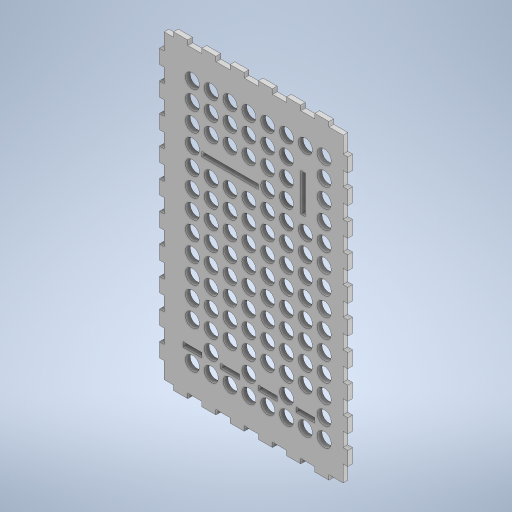
# Autodesk Inventor part: BackFrontPannel
Saved by Autodesk Inventor 2023 (Build 270158000, 158)
## iProperties
Created: 2022-09-19
Part Number: BackFrontPannel
Material: Generic
Document SubType Name: Modeling
Designer: Nathann
Density: 1 g/cm^3
Appearance: Default
Author: Nathann
Autodesk Inventor part; units mm, degrees
ref_plane "YZ Plane" through (0, 0, 0) normal (1, 0, 0) x (0, 1, 0)
ref_plane "XZ Plane" through (0, 0, 0) normal (0, 1, 0) x (-1, 0, 0)
ref_plane "XY Plane" through (0, 0, 0) normal (0, 0, 1) x (1, 0, 0)
sketch "Sketch1" plane through (0, 0, 0) normal (0, 0, 1) x (1, 0, 0)
  line L0 (0, 0) -> (200, 0)
  line L1 (200, 0) -> (200, -330)
  line L2 (200, -330) -> (0, -330)
  line L3 (0, -330) -> (0, 0)
  dimension "d0" = 200
  dimension "d1" = 330
  constraints: 8 end point, 2 parallel, 1 horizontal, 1 perpendicular
  measures "d0" distance of L0.start L0.end
  measures "d1" distance of L2.end L0.start
extrude "Extrusion1" add sketch "Sketch1" along normal blind 5
sketch "Sketch2" plane through (0, 0, 0) normal (0, 0, -1) x (-1, 0, 0)
  line L0 (0, 0) -> (-5, 0)
  line L1 (-5, 0) -> (-5, -22.5)
  line L2 (-5, -22.5) -> (0, -22.5)
  line L3 (0, -22.5) -> (0, 0)
  line L4 (-200, 0) -> (0, 0) projected
  line L5 (0, 0) -> (0, -330) projected
  line L6 (0, -37.5) -> (-5, -37.5)
  line L7 (-5, -37.5) -> (-5, -52.5)
  line L8 (-5, -52.5) -> (0, -52.5)
  line L9 (0, -52.5) -> (0, -37.5)
  line L10 (0, -30) -> (-5, -30)
  line L11 (0, -67.5) -> (-5, -67.5)
  line L12 (-5, -67.5) -> (-5, -82.5)
  line L13 (-5, -82.5) -> (0, -82.5)
  line L14 (0, -82.5) -> (0, -67.5)
  line L15 (0, -60) -> (-5, -60)
  line L16 (0, -97.5) -> (-5, -97.5)
  line L17 (-5, -97.5) -> (-5, -112.5)
  line L18 (-5, -112.5) -> (0, -112.5)
  line L19 (0, -112.5) -> (0, -97.5)
  line L20 (0, -90) -> (-5, -90)
  line L21 (0, -127.5) -> (-5, -127.5)
  line L22 (-5, -127.5) -> (-5, -142.5)
  line L23 (-5, -142.5) -> (0, -142.5)
  line L24 (0, -142.5) -> (0, -127.5)
  line L25 (0, -120) -> (-5, -120)
  line L26 (0, -157.5) -> (-5, -157.5)
  line L27 (-5, -157.5) -> (-5, -172.5)
  line L28 (-5, -172.5) -> (0, -172.5)
  line L29 (0, -172.5) -> (0, -157.5)
  line L30 (0, -150) -> (-5, -150)
  line L31 (0, -187.5) -> (-5, -187.5)
  line L32 (-5, -187.5) -> (-5, -202.5)
  line L33 (-5, -202.5) -> (0, -202.5)
  line L34 (0, -202.5) -> (0, -187.5)
  line L35 (0, -180) -> (-5, -180)
  line L36 (0, -217.5) -> (-5, -217.5)
  line L37 (-5, -217.5) -> (-5, -232.5)
  line L38 (-5, -232.5) -> (0, -232.5)
  line L39 (0, -232.5) -> (0, -217.5)
  line L40 (0, -210) -> (-5, -210)
  line L41 (0, -247.5) -> (-5, -247.5)
  line L42 (-5, -247.5) -> (-5, -262.5)
  line L43 (-5, -262.5) -> (0, -262.5)
  line L44 (0, -262.5) -> (0, -247.5)
  line L45 (0, -330) -> (-5, -330)
  line L46 (-5, -330) -> (-5, -307.5)
  line L47 (-5, -307.5) -> (0, -307.5)
  line L48 (0, -307.5) -> (0, -330)
  line L49 (-200, 0) -> (0, 0) projected
  line L50 (-100, 0) -> (-100, -60)
  line L51 (-200, 0) -> (-195, 0)
  line L52 (-195, 0) -> (-195, -22.5)
  line L53 (-195, -22.5) -> (-200, -22.5)
  line L54 (-200, -22.5) -> (-200, 0)
  line L55 (0, 0) -> (-200, 0)
  line L56 (-200, 0) -> (-200, -330)
  line L57 (-200, -37.5) -> (-195, -37.5)
  line L58 (-195, -37.5) -> (-195, -52.5)
  line L59 (-195, -52.5) -> (-200, -52.5)
  line L60 (-200, -52.5) -> (-200, -37.5)
  line L61 (-200, -30) -> (-195, -30)
  line L62 (-200, -67.5) -> (-195, -67.5)
  line L63 (-195, -67.5) -> (-195, -82.5)
  line L64 (-195, -82.5) -> (-200, -82.5)
  line L65 (-200, -82.5) -> (-200, -67.5)
  line L66 (-200, -60) -> (-195, -60)
  line L67 (-200, -97.5) -> (-195, -97.5)
  line L68 (-195, -97.5) -> (-195, -112.5)
  line L69 (-195, -112.5) -> (-200, -112.5)
  line L70 (-200, -112.5) -> (-200, -97.5)
  line L71 (-200, -90) -> (-195, -90)
  line L72 (-200, -127.5) -> (-195, -127.5)
  line L73 (-195, -127.5) -> (-195, -142.5)
  line L74 (-195, -142.5) -> (-200, -142.5)
  line L75 (-200, -142.5) -> (-200, -127.5)
  line L76 (-200, -120) -> (-195, -120)
  line L77 (-200, -157.5) -> (-195, -157.5)
  line L78 (-195, -157.5) -> (-195, -172.5)
  line L79 (-195, -172.5) -> (-200, -172.5)
  line L80 (-200, -172.5) -> (-200, -157.5)
  line L81 (-200, -150) -> (-195, -150)
  line L82 (-200, -187.5) -> (-195, -187.5)
  line L83 (-195, -187.5) -> (-195, -202.5)
  line L84 (-195, -202.5) -> (-200, -202.5)
  line L85 (-200, -202.5) -> (-200, -187.5)
  line L86 (-200, -180) -> (-195, -180)
  line L87 (-200, -217.5) -> (-195, -217.5)
  line L88 (-195, -217.5) -> (-195, -232.5)
  line L89 (-195, -232.5) -> (-200, -232.5)
  line L90 (-200, -232.5) -> (-200, -217.5)
  line L91 (-200, -210) -> (-195, -210)
  line L92 (-200, -247.5) -> (-195, -247.5)
  line L93 (-195, -247.5) -> (-195, -262.5)
  line L94 (-195, -262.5) -> (-200, -262.5)
  line L95 (-200, -262.5) -> (-200, -247.5)
  line L96 (-200, -330) -> (-195, -330)
  line L97 (-195, -330) -> (-195, -307.5)
  line L98 (-195, -307.5) -> (-200, -307.5)
  line L99 (-200, -307.5) -> (-200, -330)
  line L100 (0, 0) -> (-200, 0)
  line L101 (0, -240) -> (-5, -240)
  line L102 (0, -277.5) -> (-5, -277.5)
  line L103 (-5, -277.5) -> (-5, -292.5)
  line L104 (-5, -292.5) -> (0, -292.5)
  line L105 (0, -292.5) -> (0, -277.5)
  line L106 (-200, -277.5) -> (-195, -277.5)
  line L107 (-195, -277.5) -> (-195, -292.5)
  line L108 (-195, -292.5) -> (-200, -292.5)
  line L109 (-200, -292.5) -> (-200, -277.5)
  point P0 (0, -307.5)
  point P1 (-200, -187.5)
  point P2 (-200, -202.5)
  point P3 (0, -262.5)
  point P4 (0, -232.5)
  point P5 (0, -202.5)
  point P6 (-200, -82.5)
  point P7 (0, -172.5)
  point P8 (-200, -157.5)
  point P9 (-200, -172.5)
  point P10 (0, -142.5)
  point P11 (-200, -142.5)
  point P12 (0, -112.5)
  point P13 (-200, -97.5)
  point P14 (-200, -112.5)
  point P15 (0, -82.5)
  point P16 (-200, -247.5)
  point P17 (-200, -262.5)
  point P18 (-200, -22.5)
  point P19 (-195, 0)
  point P20 (-200, -232.5)
  point P21 (0, -292.5)
  point P22 (-200, -277.5)
  point P23 (-200, -292.5)
  dimension "d4" = 0
  dimension "d5" = 5
  dimension "d6" = 0
  dimension "d7" = 22.5
  dimension "d8" = 5
  dimension "d9" = 15
  dimension "d10" = 15
  dimension "d13" = 30
  dimension "d18" = 22.5
  dimension "d19" = 5
  constraints: 212 end point, 60 symmetric about line, 48 vertical alignment, 30 parallel, 16 collinear, 3 horizontal, 3 perpendicular, 1 midpoint, 1 vertical, 6 other
  measures "d4" distance between parallel lines of L4 L0
  measures "d5" distance of L1.end L2.end
  measures "d6" horizontal extent of L3
  measures "d7" distance of L0.end L1.end
  measures "d8" distance of L6.start L6.end
  measures "d9" distance of L6.end L7.end
  measures "d10" distance between parallel lines of L6 L2
  measures "d13" distance of L0.start L10.start
  measures "d18" distance of L45.end L46.end
  measures "d19" distance of L46.end L47.end
extrude "Extrusion2" cut sketch "Sketch2" against normal mid plane 20
sketch "Sketch6" plane through (0, 0, 0) normal (0, 0, -1) x (-1, 0, 0)
  line L0 (0, 0) -> (-15, 0)
  line L1 (-15, 0) -> (-15, -5)
  line L2 (-15, -5) -> (0, -5)
  line L3 (0, -5) -> (0, 0)
  line L4 (-30, 0) -> (-45, 0)
  line L5 (-45, 0) -> (-45, -5)
  line L6 (-45, -5) -> (-30, -5)
  line L7 (-30, -5) -> (-30, 0)
  line L8 (-60, 0) -> (-75, 0)
  line L9 (-75, 0) -> (-75, -5)
  line L10 (-75, -5) -> (-60, -5)
  line L11 (-60, -5) -> (-60, 0)
  line L12 (-90, 0) -> (-105, 0)
  line L13 (-105, 0) -> (-105, -5)
  line L14 (-105, -5) -> (-90, -5)
  line L15 (-90, -5) -> (-90, 0)
  line L16 (-120, 0) -> (-135, 0)
  line L17 (-135, 0) -> (-135, -5)
  line L18 (-135, -5) -> (-120, -5)
  line L19 (-120, -5) -> (-120, 0)
  line L20 (-150, 0) -> (-165, 0)
  line L21 (-165, 0) -> (-165, -5)
  line L22 (-165, -5) -> (-150, -5)
  line L23 (-150, -5) -> (-150, 0)
  line L24 (-180, 0) -> (-195, 0)
  line L25 (-195, 0) -> (-195, -5)
  line L26 (-195, -5) -> (-180, -5)
  line L27 (-180, -5) -> (-180, 0)
  line L28 (-195, -330) -> (-180, -330)
  line L29 (-180, -330) -> (-180, -325)
  line L30 (-180, -325) -> (-195, -325)
  line L31 (-195, -325) -> (-195, -330)
  line L32 (-150, -325) -> (-165, -325)
  line L33 (-150, -330) -> (-150, -325)
  line L34 (-165, -330) -> (-150, -330)
  line L35 (-165, -325) -> (-165, -330)
  line L36 (-120, -325) -> (-135, -325)
  line L37 (-120, -330) -> (-120, -325)
  line L38 (-135, -330) -> (-120, -330)
  line L39 (-135, -325) -> (-135, -330)
  line L40 (-90, -325) -> (-105, -325)
  line L41 (-90, -330) -> (-90, -325)
  line L42 (-105, -330) -> (-90, -330)
  line L43 (-105, -325) -> (-105, -330)
  line L44 (-60, -325) -> (-75, -325)
  line L45 (-60, -330) -> (-60, -325)
  line L46 (-75, -330) -> (-60, -330)
  line L47 (-75, -325) -> (-75, -330)
  line L48 (-30, -325) -> (-45, -325)
  line L49 (-30, -330) -> (-30, -325)
  line L50 (-45, -330) -> (-30, -330)
  line L51 (-45, -325) -> (-45, -330)
  line L52 (0, -325) -> (-15, -325)
  line L53 (0, -330) -> (0, -325)
  line L54 (-15, -330) -> (0, -330)
  line L55 (-15, -325) -> (-15, -330)
  line L56 (-155, -60) -> (-155, -100) projected
  line L57 (-150, -60) -> (-150, -100) projected
  line L58 (-155, -60) -> (-150, -60) projected
  line L59 (-155, -100) -> (-150, -100) projected
  line L60 (-105, -100) -> (-45, -100) projected
  line L61 (-105, -95) -> (-45, -95) projected
  line L62 (-105, -95) -> (-105, -100) projected
  line L63 (-45, -100) -> (-45, -95) projected
  line L64 (-45, -285) -> (-25, -285) projected
  line L65 (-45, -280) -> (-25, -280) projected
  line L66 (-25, -285) -> (-25, -280) projected
  line L67 (-45, -280) -> (-45, -285) projected
  line L68 (-85, -285) -> (-65, -285) projected
  line L69 (-85, -280) -> (-65, -280) projected
  line L70 (-65, -285) -> (-65, -280) projected
  line L71 (-85, -280) -> (-85, -285) projected
  line L72 (-125, -285) -> (-105, -285) projected
  line L73 (-125, -280) -> (-105, -280) projected
  line L74 (-105, -285) -> (-105, -280) projected
  line L75 (-125, -280) -> (-125, -285) projected
  line L76 (-165, -285) -> (-145, -285) projected
  line L77 (-165, -280) -> (-145, -280) projected
  line L78 (-145, -285) -> (-145, -280) projected
  line L79 (-165, -280) -> (-165, -285) projected
  dimension "d70" = 5
  dimension "d71" = 15
  dimension "d74" = 30
  dimension "d79" = 5
  dimension "d80" = 15
  dimension "d83" = 30
  constraints: 112 end point, 4 horizontal, 4 parallel, 2 collinear, 2 perpendicular, 94 other
  measures "d70" distance of L0.end L1.end
  measures "d71" distance of L1.end L2.end
  measures "d74" distance of L1.end L5.end
  measures "d79" distance between parallel lines of L28 L30
  measures "d80" distance of L29.end L30.end
  measures "d83" distance of L29.end L32.start
extrude "Extrusion6" cut sketch "Sketch6" against normal blind 10
sketch "Sketch7" plane through (0, 0, 5) normal (0, 0, 1) x (1, 0, 0)
  circle A0 centre (35, -35) radius 7.5
  line L0 (45, -5) -> (30, -5) projected
  line L1 (5, -5) -> (5, -22.5) projected
  circle A1 centre (35, -55) radius 7.5
  circle A2 centre (35, -75) radius 7.5
  circle A3 centre (35, -95) radius 7.5
  circle A4 centre (35, -115) radius 7.5
  circle A5 centre (35, -135) radius 7.5
  circle A6 centre (35, -155) radius 7.5
  circle A7 centre (35, -175) radius 7.5
  circle A8 centre (35, -195) radius 7.5
  circle A9 centre (35, -215) radius 7.5
  circle A10 centre (35, -235) radius 7.5
  circle A11 centre (35, -255) radius 7.5
  circle A12 centre (35, -275) radius 7.5
  circle A13 centre (35, -295) radius 7.5
  circle A14 centre (55, -35) radius 7.5
  circle A15 centre (55, -55) radius 7.5
  circle A16 centre (55, -75) radius 7.5
  circle A17 centre (55, -95) radius 7.5
  circle A18 centre (55, -115) radius 7.5
  circle A19 centre (55, -135) radius 7.5
  circle A20 centre (55, -155) radius 7.5
  circle A21 centre (55, -175) radius 7.5
  circle A22 centre (55, -195) radius 7.5
  circle A23 centre (55, -215) radius 7.5
  circle A24 centre (55, -235) radius 7.5
  circle A25 centre (55, -255) radius 7.5
  circle A26 centre (55, -275) radius 7.5
  circle A27 centre (55, -295) radius 7.5
  circle A28 centre (75, -35) radius 7.5
  circle A29 centre (75, -55) radius 7.5
  circle A30 centre (75, -75) radius 7.5
  circle A31 centre (75, -95) radius 7.5
  circle A32 centre (75, -115) radius 7.5
  circle A33 centre (75, -135) radius 7.5
  circle A34 centre (75, -155) radius 7.5
  circle A35 centre (75, -175) radius 7.5
  circle A36 centre (75, -195) radius 7.5
  circle A37 centre (75, -215) radius 7.5
  circle A38 centre (75, -235) radius 7.5
  circle A39 centre (75, -255) radius 7.5
  circle A40 centre (75, -275) radius 7.5
  circle A41 centre (75, -295) radius 7.5
  circle A42 centre (95, -35) radius 7.5
  circle A43 centre (95, -55) radius 7.5
  circle A44 centre (95, -75) radius 7.5
  circle A45 centre (95, -95) radius 7.5
  circle A46 centre (95, -115) radius 7.5
  circle A47 centre (95, -135) radius 7.5
  circle A48 centre (95, -155) radius 7.5
  circle A49 centre (95, -175) radius 7.5
  circle A50 centre (95, -195) radius 7.5
  circle A51 centre (95, -215) radius 7.5
  circle A52 centre (95, -235) radius 7.5
  circle A53 centre (95, -255) radius 7.5
  circle A54 centre (95, -275) radius 7.5
  circle A55 centre (95, -295) radius 7.5
  circle A56 centre (115, -35) radius 7.5
  circle A57 centre (115, -55) radius 7.5
  circle A58 centre (115, -75) radius 7.5
  circle A59 centre (115, -95) radius 7.5
  circle A60 centre (115, -115) radius 7.5
  circle A61 centre (115, -135) radius 7.5
  circle A62 centre (115, -155) radius 7.5
  circle A63 centre (115, -175) radius 7.5
  circle A64 centre (115, -195) radius 7.5
  circle A65 centre (115, -215) radius 7.5
  circle A66 centre (115, -235) radius 7.5
  circle A67 centre (115, -255) radius 7.5
  circle A68 centre (115, -275) radius 7.5
  circle A69 centre (115, -295) radius 7.5
  circle A70 centre (135, -35) radius 7.5
  circle A71 centre (135, -55) radius 7.5
  circle A72 centre (135, -75) radius 7.5
  circle A73 centre (135, -95) radius 7.5
  circle A74 centre (135, -115) radius 7.5
  circle A75 centre (135, -135) radius 7.5
  circle A76 centre (135, -155) radius 7.5
  circle A77 centre (135, -175) radius 7.5
  circle A78 centre (135, -195) radius 7.5
  circle A79 centre (135, -215) radius 7.5
  circle A80 centre (135, -235) radius 7.5
  circle A81 centre (135, -255) radius 7.5
  circle A82 centre (135, -275) radius 7.5
  circle A83 centre (135, -295) radius 7.5
  circle A84 centre (155, -35) radius 7.5
  circle A85 centre (155, -55) radius 7.5
  circle A86 centre (155, -75) radius 7.5
  circle A87 centre (155, -95) radius 7.5
  circle A88 centre (155, -115) radius 7.5
  circle A89 centre (155, -135) radius 7.5
  circle A90 centre (155, -155) radius 7.5
  circle A91 centre (155, -175) radius 7.5
  circle A92 centre (155, -195) radius 7.5
  circle A93 centre (155, -215) radius 7.5
  circle A94 centre (155, -235) radius 7.5
  circle A95 centre (155, -255) radius 7.5
  circle A96 centre (155, -275) radius 7.5
  circle A97 centre (155, -295) radius 7.5
  circle A98 centre (175, -35) radius 7.5
  circle A99 centre (175, -55) radius 7.5
  circle A100 centre (175, -75) radius 7.5
  circle A101 centre (175, -95) radius 7.5
  circle A102 centre (175, -115) radius 7.5
  circle A103 centre (175, -135) radius 7.5
  circle A104 centre (175, -155) radius 7.5
  circle A105 centre (175, -175) radius 7.5
  circle A106 centre (175, -195) radius 7.5
  circle A107 centre (175, -215) radius 7.5
  circle A108 centre (175, -235) radius 7.5
  circle A109 centre (175, -255) radius 7.5
  circle A110 centre (175, -275) radius 7.5
  circle A111 centre (175, -295) radius 7.5
  point P0 (0, 0)
  dimension "d90" = 30
  dimension "d91" = 30
  dimension "d92" = 15
  dimension "d95" = 20
  dimension "d98" = 20
  constraints: 112 centre point, 1 horizontal, 1 vertical, 222 other
  measures "d90" distance from line of A0.centre L0
  measures "d91" distance from line of L1 A0.centre
  measures "d92" diameter of A0
  measures "d95" distance of A0.centre A1.centre
  measures "d98" distance of A0.centre A14.centre
extrude "Extrusion7" cut sketch "Sketch7" against normal blind 10 contours A0 | A1 | A2 | A3 | A4 | A5 | A6 | A7 | A8 | A9 | A10 | A11 | A13 | A14 | A15 | A16 | A18 | A19 | A20 | A21 | A22 | A23 | A24 | A25 | A26 | A27 | A28 | A29 | A30 | A32 | A33 | A34 | A35 | A36 | A37 | A38 | A39 | A41 | A42 | A43 | A44 | A46 | A47 | A48 | A49 | A50 | A51 | A52 | A53 | A54 | A55 | A56 | A57 | A58 | A59 | A60 | A61 | A62 | A63 | A64 | A65 | A66 | A67 | A69 | A70 | A71 | A72 | A73 | A74 | A75 | A76 | A77 | A78 | A79 | A80 | A81 | A82 | A83 | A84 | A88 | A89 | A90 | A91 | A92 | A93 | A94 | A95 | A97 | A98 | A99 | A100 | A101 | A102 | A103 | A104 | A105 | A106 | A107 | A108 | A109 | A110 | A111
equation "\"d2\" = WoodWidth"
equation "\"d5\" = WoodWidth - LaserWith"
equation "\"d8\" = d5"
equation "\"d18\" = d7"
equation "\"d19\" = d5"
equation "\"d20\" = 4 * WoodWidth"
equation "\"d90\" = d91"
equation "\"WoodWidth\" = 5"
equation "\"LaserWith\" = 0"
body "Solid1"
